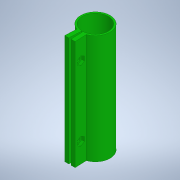
# Autodesk Inventor part: X-Motor P1
Saved by Autodesk Inventor 2020 (Build 240168000, 168)
## iProperties
Created: 2019-09-14
Part Number: X-Motor P1
Material: Generic
Document SubType Name: Modeling
Designer: pepd9
Density: 1 g/cm^3
Appearance: Dark Green
Author: pepd9
Autodesk Inventor part; units mm, degrees
note: some values were not read from the file. Chosen so that the rebuilt part matches the saved one: direction of "Hole1".
ref_plane "YZ Plane" through (0, 0, 0) normal (1, 0, 0) x (0, 1, 0)
ref_plane "XZ Plane" through (0, 0, 0) normal (0, 1, 0) x (-1, 0, 0)
ref_plane "XY Plane" through (0, 0, 0) normal (0, 0, 1) x (1, 0, 0)
sketch "Sketch1" plane through (0, 0, 0) normal (0, 1, 0) x (-1, 0, 0)
  arc A0 (-0.4144, 9.491) -> (0.4144, 9.491) centre (0, 0) ccw
  arc A1 (-0.4667, 10.6898) -> (0.4667, 10.6898) centre (0, 0) ccw
  line L0 (0, 0) -> (-0.4667, 10.6898)
  line L1 (0, 0) -> (0.4667, 10.6898)
  line L2 (0, 0) -> (0, 8.5605) construction
  dimension "d0" = 19
  dimension "d1" = 21.4
  dimension "d2" = 5
  dimension "d3" = 2.5
  constraints: 6 end point, 4 point on circle, 2 centre point, 2 coincident, 2 point on line, 1 vertical
  measures "d0" diameter of A0
  measures "d1" diameter of A1
  measures "d2" angle of L0 L1
  measures "d3" angle of L2 L0
extrude "BearingSleeve" add sketch "Sketch1" along normal blind 80 contours A0 L1 A1 L0
sketch "Sketch2" plane through (0, 80, 0) normal (0, 1, 0) x (1, 0, 0)
  arc A0 (0.4144, -9.491) -> (-0.4144, -9.491) centre (0, 0) ccw projected
  line L0 (-0.4144, -9.491) -> (-0.816, -18.6898)
  line L1 (0.4144, -9.491) -> (0.816, -18.6898)
  line L2 (-0.4667, -10.6898) -> (-0.4144, -9.491) projected
  line L3 (0.4144, -9.491) -> (0.4667, -10.6898) projected
  line L4 (3.3903, -8.8744) -> (3.8189, -18.6898)
  line L5 (-3.3903, -8.8744) -> (-3.8189, -18.6898)
  line L6 (-3.8189, -18.6898) -> (-0.816, -18.6898)
  line L7 (0.816, -18.6898) -> (3.8189, -18.6898)
  dimension "d6" = 3
  dimension "d7" = 3
  dimension "d8" = 8
  dimension "d9" = 8
  constraints: 12 end point, 2 horizontal alignment, 2 parallel, 2 point on circle, 2 point on line, 1 collinear, 1 horizontal
  measures "d6" distance between parallel lines of L4 L1
  measures "d7" distance between parallel lines of L5 L0
  measures "d8" vertical distance of L3.end L1.end
  measures "d9" vertical distance of L2.start L0.end
extrude "BearingLocks" add sketch "Sketch2" against normal up to surface (80 mm away)
sketch "Sketch3" plane through (-3.4452, 0, 10.1302) normal (-0.9990482, 0, -0.0436194) x (-0.0436194, 0, 0.9990482)
  line L0 (8.5678, 0) -> (0, 0) projected
  line L1 (0, 80) -> (8.5678, 80) projected
  line L2 (8.5678, 80) -> (8.5678, 0) projected
  point P0 (-10.2708, 0)
  point P1 (4.1678, 14.5)
  point P2 (4.1678, 65.5)
  dimension "d12" = 14.5
  dimension "d13" = 14.5
  dimension "d14" = 4.4
  dimension "d15" = 4.4
  measures "d12" distance from line of L0 point (4.168, 14.5)
  measures "d13" distance from line of L1 point (4.168, 65.5)
  measures "d14" distance from line of L2 point (4.168, 65.5)
  measures "d15" distance from line of L2 point (4.168, 14.5)
hole "Hole1" at (-3.6269, 14.5, 14.294) at (-3.6269, 65.5, 14.294) direction (0.9990482, 0, 0.0436194) diameter 3.6 end up to surface counterbore diameter 6.5 counterbore depth 1.5 clearance for "Socket Head Cap Screw" size "M3" standard "Ansi Metric M Profile"
sketch "Sketch4" plane through (3.4452, 0, 10.1302) normal (0.9990482, 0, -0.0436194) x (-0.0436194, 0, -0.9990482)
  line L0 (-8.5678, 80) -> (0, 80) projected
  line L1 (0, 0) -> (-8.5678, 0) projected
  line L2 (-8.5678, 80) -> (-8.5678, 0) projected
  point P0 (10.2708, 0)
  point P1 (-4.1678, 65.5)
  point P2 (-4.1678, 14.5)
  dimension "d23" = 14.5
  dimension "d24" = 14.5
  dimension "d25" = 4.4
  dimension "d26" = 4.4
  measures "d23" distance from line of L0 point (-4.168, 65.5)
  measures "d24" distance from line of L1 point (-4.168, 14.5)
  measures "d25" distance from line of L2 point (-4.168, 14.5)
  measures "d26" distance from line of L2 point (-4.168, 65.5)
hole "Hole2" at (3.6269, 65.5, 14.294) at (3.6269, 14.5, 14.294) direction (-0.9990482, 0, 0.0436194) diameter 3.4 depth 3 clearance for "Socket Head Cap Screw" size "M3" standard "Ansi Metric M Profile"
sketch "Sketch5" plane through (3.4452, 0, 10.1302) normal (0.9990482, 0, -0.0436194) x (-0.0436194, 0, -0.9990482)
  circle A0 centre (-4.1678, 65.5) radius 1.7 projected
  circle A1 centre (-4.1678, 14.5) radius 1.7 projected
  line L0 (0, 80) -> (0, 0) projected
  line L1 (-8.5678, 80) -> (0, 80) projected
  line L2 (-8.5678, 80) -> (-8.5678, 0) projected
  line L3 (0, 0) -> (-8.5678, 0) projected
  line L4 (-1.4178, 12.9123) -> (-4.1678, 11.3246)
  line L5 (-4.1678, 11.3246) -> (-6.9178, 12.9123)
  line L6 (-6.9178, 12.9123) -> (-6.9178, 16.0877)
  line L7 (-6.9178, 16.0877) -> (-4.1678, 17.6754)
  line L8 (-4.1678, 17.6754) -> (-1.4178, 16.0877)
  line L9 (-1.4178, 16.0877) -> (-1.4178, 12.9123)
  line L10 (-1.4178, 63.9123) -> (-4.1678, 62.3246)
  line L11 (-4.1678, 62.3246) -> (-6.9178, 63.9123)
  line L12 (-6.9178, 63.9123) -> (-6.9178, 67.0877)
  line L13 (-6.9178, 67.0877) -> (-4.1678, 68.6754)
  line L14 (-4.1678, 68.6754) -> (-1.4178, 67.0877)
  line L15 (-1.4178, 67.0877) -> (-1.4178, 63.9123)
  point P0 (10.2708, 0)
  dimension "d34" = 5.5
  dimension "d35" = 5.5
  constraints: 24 end point, 2 coincident, 26 other
  measures "d34" distance between parallel lines of L15 L12
  measures "d35" distance between parallel lines of L9 L6
extrude "Extrusion3" cut sketch "Sketch5" against normal blind 2 contours L4 L5 L6 L7 L8 L9 | L10 L11 L12 L13 L14 L15
equation "\"d0\" = BearingOD"
equation "\"d1\" = BearingOD + BearingClampWallThickness"
equation "\"d2\" = BearingTensionGap"
equation "\"d3\" = 0.5 * BearingTensionGap"
equation "\"d4\" = EffectiveBearingLength"
equation "\"d10\" = EffectiveBearingLength"
equation "\"d12\" = 0.5 * BearingLength"
equation "\"d13\" = 0.5 * BearingLength"
equation "\"d23\" = 0.5 * BearingLength"
equation "\"d24\" = 0.5 * BearingLength"
equation "\"BearingOD\" = 19"
equation "\"NozzleDiameter\" = 0.4"
equation "\"BearingTensionGap\" = 5deg"
equation "\"BearingLength\" = 29"
equation "\"EffectiveBearingLength\" = 80"
equation "\"BearingSpacing\" = EffectiveBearingLength - 2 * BearingLength"
equation "\"BearingClampWallThickness\" = 6 * NozzleDiameter"
equation "\"BearingClampLength\" = 8"
body "Solid1"
